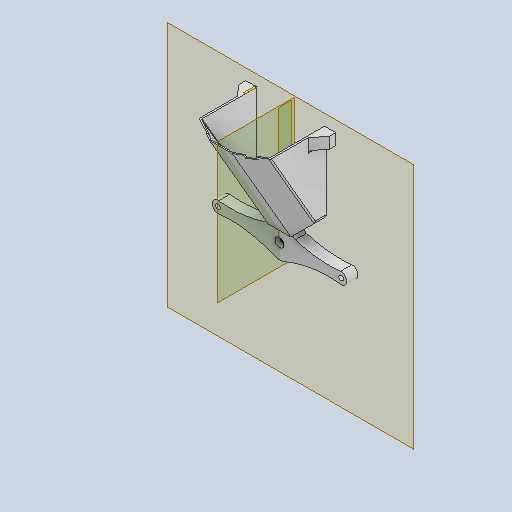
# Autodesk Inventor part: Brida_Rodamiento_Inferior
Saved by Autodesk Inventor 2024 (Build 280153000, 153)
## iProperties
Created: 2024-07-16
Part Number: Brida_Rodamiento_Inferior
Material: Genérico
Document SubType Name: Modeling
Designer: sergi
Density: 1 g/cm^3
Appearance: Valor por defecto
Author: sergi
Autodesk Inventor part; units mm, degrees
ref_plane "YZ Plane" through (0, 0, 0) normal (1, 0, 0) x (0, 1, 0)
ref_plane "XZ Plane" through (0, 0, 0) normal (0, 1, 0) x (-1, 0, 0)
ref_plane "XY Plane" through (0, 0, 0) normal (0, 0, 1) x (1, 0, 0)
sketch "Boceto1" plane through (0, 0, 0) normal (0, 0, 1) x (1, 0, 0)
  circle A0 centre (0, 0) radius 8.25 projected
  arc A1 (-36.7643, -25.9497) -> (36.7643, -25.9497) centre (0, 0) ccw projected
  arc A2 (-35.5756, -20.5396) -> (-36.7643, -25.9497) centre (-33.7006, -23.7872) ccw projected
  line L0 (-35.5756, -20.5396) -> (-15.9099, -9.1856) projected
  arc A3 (-11.2279, -9.9465) -> (-15.9099, -9.1856) centre (-14.0349, -12.4332) ccw projected
  arc A4 (-11.2279, -9.9465) -> (11.2279, -9.9465) centre (0, 0) ccw projected
  arc A5 (15.9099, -9.1856) -> (11.2279, -9.9465) centre (14.0349, -12.4332) ccw projected
  line L1 (15.9099, -9.1856) -> (35.5756, -20.5396) projected
  arc A6 (36.7643, -25.9497) -> (35.5756, -20.5396) centre (33.7006, -23.7872) ccw projected
  line L2 (98, -98) -> (98, 98) projected
  line L3 (98, 98) -> (-98, 98) projected
  line L4 (-98, 98) -> (-98, -98) projected
  line L5 (-98, -98) -> (98, -98) projected
  circle A7 centre (0, 0) radius 4 projected
  line L6 (21.4655, -12.3931) -> (15.9099, -9.1856) projected
  arc A8 (15.9099, -9.1856) -> (11.2279, -9.9465) centre (14.0349, -12.4332) ccw projected
  arc A9 (-11.2279, -9.9465) -> (11.2279, -9.9465) centre (0, 0) ccw projected
  arc A10 (-11.2279, -9.9465) -> (-15.9099, -9.1856) centre (-14.0349, -12.4332) ccw projected
  line L7 (-15.9099, -9.1856) -> (-21.4655, -12.3931) projected
  line L8 (0, 0) -> (-55, 0) construction
  line L9 (0, 0) -> (55, 0) construction
  circle A11 centre (-55, 0) radius 2.1
  circle A12 centre (0, 0) radius 4
  circle A13 centre (-55, 0) radius 5
  circle A14 centre (0, 0) radius 13.4
  circle A15 centre (44.1778, -104.4408) radius 100
  circle A16 centre (-44.1778, -104.4408) radius 100
  arc A17 (0, 14.7284) -> (-5.2203, 12.3413) centre (-44.1778, 104.4408) ccw
  arc A18 (5.2203, 12.3413) -> (0, 14.7284) centre (44.1778, 104.4408) ccw
  line L10 (0, 0) -> (55, 0) construction
  circle A19 centre (55, 0) radius 5
  circle A20 centre (55, 0) radius 2.1
  line L11 (21.4655, -12.3931) -> (21.4655, 21.4655) projected
  line L12 (-21.4655, 21.4655) -> (-21.4655, -12.3931) projected
  line L13 (21.4655, 21.4655) -> (-21.4655, 21.4655) projected
  line L14 (-5.2203, 12.3413) -> (5.2203, 12.3413)
  line L15 (-11.6313, 9.8854) -> (11.6313, 9.8854)
  point P0 (0, 0)
  point P1 (21.8181, -12.5967)
  point P2 (-21.8181, -12.5967)
  point P3 (-11.6313, -9.4678)
  point P4 (-6.1957, 13.6607)
  point P5 (-54.4847, 4.9734)
  point P6 (-54.4847, -4.9734)
  point P7 (-14.9695, -8.8015)
  point P8 (14.9695, -8.8015)
  point P9 (6.1957, 13.6607)
  point P10 (27.9997, -35.2281)
  point P11 (-27.9997, -35.2281)
  point P12 (-11.1255, -10.061)
  point P13 (11.1255, -10.061)
  point P14 (11.2279, -9.9465)
  point P15 (11.2279, -9.9465)
  point P16 (54.4847, -4.9734)
  point P17 (54.4847, 4.9734)
  point P18 (25.5998, 0)
  point P19 (43.9457, 0)
  point P20 (-43.9457, 0)
  point P21 (-25.5998, 0)
  point P22 (-5.2203, -12.3413)
  point P23 (5.2203, -12.3413)
  point P24 (0, 192.7304)
  point P25 (0, 194.1532)
  point P26 (0, -194.1532)
  point P27 (0, -14.7284)
  point P28 (0.5287, -14.9907)
  point P29 (-0.5287, -14.9907)
  dimension "d3" = 180
  dimension "d4" = 4.2
  dimension "d16" = 10
  dimension "d18" = 55
  dimension "d19" = 26.8
  dimension "empalme" = 200
  dimension "d22" = 200
  dimension "d23" = 200
  dimension "d24" = 200
  dimension "d27" = 55
  dimension "d28" = 10
  dimension "d29" = 4.2
  constraints: 10 centre point, 10 end point, 8 point on circle, 8 tangent, 6 coincident, 3 horizontal, 1 collinear, 1 concentric, 1 point on line
  measures "d3" angle of L8 L9
  measures "d4" diameter of A11
  measures "d16" diameter of A13
  measures "d18" distance of L8.start L8.end
  measures "d19" diameter of A14
  measures "empalme" diameter of A15
  measures "d22" diameter of A16
  measures "d23" diameter of A17
  measures "d24" diameter of A18
  measures "d27" distance of L10.start L10.end
  measures "d28" diameter of A19
  measures "d29" diameter of A20
extrude "Extrusión1" add sketch "Boceto1" along normal blind 10 contours A0 | A16 A3 A4 | A4 A3 A16 L12 A17 L15 A14 | A16 A13 A17 L12 | A15 A14 L15 A18 L11 A5 A4 | A4 A5 A15 | A14 L15 | A13 | L11 A18 A19 A15 | A19
sketch "Boceto2" plane through (0, 0, 0) normal (0, 0, -1) x (-1, 0, 0)
  circle A0 centre (0, 0) radius 8.25 projected
  point P0 (0, 0)
extrude "Extrusión2" cut sketch "Boceto2" against normal blind 5
sketch "Boceto3" plane through (0, 0, 5) normal (0, 0, -1) x (-1, 0, 0)
  circle A0 centre (0, 0) radius 5.25 projected
  point P0 (0, 0)
extrude "Extrusión3" cut sketch "Boceto3" against normal blind 0.5
ref_plane "Plano de trabajo1" through (0, 0, 0) normal (0, 0, 1) x (1, 0, 0)
sketch "Boceto4" plane through (0, 0, 0) normal (0, 0, 1) x (1, 0, 0)
  line L0 (-31.8102, 100) -> (-31.8102, 32.4528) projected
  arc A0 (-31.8102, 32.4528) -> (-30.7558, 29.9072) centre (-28.2102, 32.4528) ccw projected
  line L1 (-30.7558, 29.9072) -> (-10.7339, 9.8854) projected
  line L2 (10.7339, 9.8854) -> (10.7339, 100) projected
  line L3 (30.7558, 29.9072) -> (30.7558, 100) projected
  line L4 (30.7558, 29.9072) -> (10.7339, 9.8854) projected
  line L5 (30.7558, 29.9072) -> (30.7558, 100) projected
  line L6 (-30.2102, 32.4528) -> (-30.2102, 100) projected
  arc A1 (-30.2102, 32.4528) -> (-29.6244, 31.0386) centre (-28.2102, 32.4528) ccw projected
  line L7 (-9.8759, 11.2901) -> (-29.6244, 31.0386) projected
  line L8 (9.8759, 11.2901) -> (-9.8759, 11.2901) projected
  line L9 (11.6313, 9.8854) -> (-11.6313, 9.8854) projected
  line L10 (29.6244, 31.0386) -> (9.8759, 11.2901) projected
  arc A2 (29.6244, 31.0386) -> (30.2102, 32.4528) centre (28.2102, 32.4528) ccw projected
  line L11 (30.2102, 100) -> (30.2102, 32.4528) projected
  line L12 (100, 100) -> (-100, 100) projected
  line L13 (31.8102, 32.4528) -> (31.8102, 100) projected
  arc A3 (30.7558, 29.9072) -> (31.8102, 32.4528) centre (28.2102, 32.4528) ccw projected
  line L14 (11.6313, 9.8854) -> (11.6313, 10.7827)
  line L15 (-11.6313, 9.8854) -> (-11.6313, 10.7827)
  point P0 (0, 0)
  point P1 (10.7339, 12.1481)
  constraints: 4 end point, 2 point on line, 1 parallel, 1 vertical
extrude "Extrusión4" add sketch "Boceto4" along normal up to surface (10 mm away) contours L12 L6 A1 L7 L8 L10 L2 L9 L1 A0 L0 | L1 L9 L15 | L10 A2 L11 L12 L3 L4 L2 | L4 L14 L9 | L12 L13 A3 L3
fillet "Empalme2" radius 2 4 edges at (-11.6313, 9.8854, 5) (-11.6313, 10.7827, 5) (11.6313, 9.8854, 5) (11.6313, 10.7827, 5)
sketch "Boceto5" plane through (0, 0, 10) normal (0, 0, 1) x (1, 0, 0)
  line L0 (-10.1386, 9.2901) -> (-30.7558, 29.9072)
  arc A0 (-31.8102, 32.4528) -> (-30.7558, 29.9072) centre (-28.2102, 32.4528) ccw projected
  arc A1 (-30.2102, 32.4528) -> (-29.6244, 31.0386) centre (-28.2102, 32.4528) ccw projected
  line L1 (-29.6244, 31.0386) -> (-9.8759, 11.2901) projected
  line L2 (-9.8759, 11.2901) -> (9.8759, 11.2901) projected
  line L3 (9.8759, 11.2901) -> (29.6244, 31.0386) projected
  line L4 (30.7558, 29.9072) -> (10.1386, 9.2901)
  arc A2 (30.7558, 29.9072) -> (31.8102, 32.4528) centre (28.2102, 32.4528) ccw projected
  line L5 (-103, 100) -> (100, 100) projected
  arc A3 (-54.4847, 4.9734) -> (-11.6313, 9.8854) centre (-44.1778, 104.4408) ccw projected
  arc A4 (-54.4847, 4.9734) -> (-11.6313, 9.8854) centre (-44.1778, 104.4408) ccw projected
  arc A5 (13.4151, 9.2901) -> (54.4847, 4.9734) centre (44.1778, 104.4408) ccw
  line L6 (11.6313, 10.7827) -> (11.6313, 9.8854) projected
  line L7 (-11.6313, 9.8854) -> (-11.6313, 10.7827) projected
  arc A6 (-54.4847, 4.9734) -> (-14.0645, 9.0826) centre (-44.1778, 104.4408) ccw projected
  arc A7 (-54.4847, 4.9734) -> (-54.4847, -4.9734) centre (-55, 0) ccw projected
  arc A8 (-5.2203, -12.3413) -> (-54.4847, -4.9734) centre (-44.1778, -104.4408) ccw projected
  arc A9 (-5.2203, -12.3413) -> (5.2203, -12.3413) centre (0, 0) ccw projected
  arc A10 (54.4847, -4.9734) -> (5.2203, -12.3413) centre (44.1778, -104.4408) ccw projected
  arc A11 (54.4847, -4.9734) -> (54.4847, 4.9734) centre (55, 0) ccw projected
  arc A12 (14.0645, 9.0826) -> (54.4847, 4.9734) centre (44.1778, 104.4408) ccw projected
  circle A13 centre (0, 0) radius 4 projected
  line L8 (-14.0645, 9.0826) -> (-14.0158, 9.0987)
  line L9 (0, 11.2901) -> (0, 9.2901)
  line L10 (0, 9.2901) -> (-13.4151, 9.2901)
  line L11 (0, 9.2901) -> (13.4151, 9.2901)
  line L12 (30.7558, 29.9072) -> (13.2525, 12.404) projected
  arc A14 (30.7558, 29.9072) -> (31.8102, 32.4528) centre (28.2102, 32.4528) ccw projected
  line L13 (31.8102, 100) -> (31.8102, 32.4528) projected
  line L14 (30.2102, 100) -> (31.8102, 100) projected
  line L15 (30.2102, 32.4528) -> (30.2102, 100) projected
  arc A15 (29.6244, 31.0386) -> (30.2102, 32.4528) centre (28.2102, 32.4528) ccw projected
  line L16 (9.8759, 11.2901) -> (29.6244, 31.0386) projected
  line L17 (-9.8759, 11.2901) -> (9.8759, 11.2901) projected
  line L18 (-29.6244, 31.0386) -> (-9.8759, 11.2901) projected
  arc A16 (-30.2102, 32.4528) -> (-29.6244, 31.0386) centre (-28.2102, 32.4528) ccw projected
  line L19 (-30.2102, 100) -> (-30.2102, 32.4528) projected
  line L20 (-31.8102, 100) -> (-30.2102, 100) projected
  line L21 (-31.8102, 32.4528) -> (-31.8102, 100) projected
  arc A17 (-31.8102, 32.4528) -> (-30.7558, 29.9072) centre (-28.2102, 32.4528) ccw projected
  line L22 (-13.2525, 12.404) -> (-30.7558, 29.9072) projected
  arc A18 (-14.0645, 9.0826) -> (-13.2525, 12.404) centre (-14.6667, 10.9898) ccw projected
  arc A19 (13.2525, 12.404) -> (14.0645, 9.0826) centre (14.6667, 10.9898) ccw projected
  point P0 (0, 0)
  point P1 (-31.8102, 100)
  point P2 (-30.2102, 100)
  point P3 (30.2102, 100)
  point P4 (31.8102, 100)
  point P5 (-31.8102, 32.4528)
  dimension "d59" = 2
  constraints: 12 end point, 4 point on circle, 2 point on line, 1 centre point, 1 horizontal, 1 perpendicular
  measures "d59" distance of L9.start L9.end
ref_plane "Plano de trabajo2" through (0, 32.4528, 0) normal (-1, 0, 0) x (0, 0, 1)
sketch "Boceto6" plane through (0, 32.4528, 0) normal (-1, 0, 0) x (0, 0, 1)
  line L0 (10, -23.1627) -> (81, 99.8129)
  point P0 (10, 67.5472)
  constraints: 2 end point
sweep "Barrido1" add profiles "Boceto5" path "Boceto6" keep normal constant yes contours L0 A0 L21 L5 L19 A1 L1 L2 L9 L10 | L9 L2 L3 A15 L15 L5 L13 A2 L4 L11
ref_plane "Plano de trabajo3" through (-31.8102, 100, 0) normal (0, 1, 0) x (1, 0, 0)
split "Dividir1" plane through (-31.8102, 100, 0) removes the side toward (0, 1, 0)
sketch "Boceto7" plane through (-31.8102, 32.4528, 0) normal (-1, 0, 0) x (0, 0, 1)
  line L0 (0, 67.5472) -> (48.9984, 67.5472) projected
  line L1 (0, 67.5472) -> (0, 0) projected
  line L2 (0, 0) -> (10, 0) projected
  line L3 (0, 67.5472) -> (16, 67.5472)
  line L4 (16, 67.5472) -> (16, 57.5472)
  line L5 (16, 57.5472) -> (0, 57.5472)
  line L6 (0, 57.5472) -> (0, 67.5472)
  line L7 (10, 0) -> (48.9984, 67.5472) projected
  point P0 (0, -32.4528)
  point P1 (0, 57.5472)
  point P2 (16, 67.5472)
  point P3 (16, 67.5472)
  dimension "d41" = 10
  dimension "d56" = 16
  constraints: 8 end point, 2 parallel, 1 horizontal, 1 perpendicular
  measures "d41" distance of L3.end L4.end
  measures "d56" distance of L4.end L5.end
extrude "Extrusión5" add sketch "Boceto7" along normal blind 8.4 contours L0 L4 L5 L1
chamfer "Chaflán2" distance 10 distance2 8.4 1 edges at (-40.2102, 95, 16) measured on face at (-40.2102, 95, 15.5)
sketch "Boceto8" plane through (0, 0, 0) normal (0, 0, -1) x (-1, 0, 0)
  line L0 (30.2102, 100) -> (-31.8102, 100) projected
  line L1 (30.2102, 32.4528) -> (30.2102, 100) projected
  line L2 (40.2102, 100) -> (40.2102, 90) projected
  line L3 (-98, 100) -> (100, 100) projected
  line L4 (31.8102, 90) -> (40.2102, 90) projected
  line L5 (31.8102, 90) -> (31.8102, 32.4528) projected
  circle A0 centre (35, 95) radius 2.1
  point P0 (0, 0)
  point P1 (25.2102, 95)
  point P2 (31.8102, 100)
  dimension "d47" = 5
  dimension "d55" = 5
  dimension "d62" = 4.2
  constraints: 1 centre point
  measures "d47" distance from line of L0 point (25.21, 95)
  measures "d55" distance from line of L1 point (25.21, 95)
  measures "d62" diameter of A0
hole "Agujero1" at (-35, 95, 0) direction (0, 0, 1) diameter 4.2 depth 4
ref_plane "Plano de trabajo4" through (0, 32.4528, 0) normal (-1, 0, 0) x (0, 0, 1)
mirror "Simetría1" about plane through (0, 32.4528, 0) normal (-1, 0, 0) of "Extrusión5", "Chaflán2", "Agujero1"
fillet "Empalme1" radius 2 4 edges at (-31.8102, 90, 16) (-31.8102, 90, 8) (31.8102, 90, 16) (31.8102, 90, 8)
sketch "Boceto9" plane through (-10.1386, 100, 62.3714) normal (0, 1, 0) x (1, 0, 0)
  line L0 (-89.8614, 115.3714) -> (-92.8614, 115.3714) projected
  line L1 (-92.8614, 115.3714) -> (-92.8614, 90.3714) projected
  line L2 (-92.8614, 90.3714) -> (-89.8614, 90.3714) projected
  line L3 (-89.8614, 90.3714) -> (-89.8614, 65.3714) projected
  line L4 (-89.8614, 65.3714) -> (-92.8614, 65.3714) projected
  line L5 (-92.8614, 65.3714) -> (-92.8614, 40.3714) projected
  line L6 (-92.8614, 40.3714) -> (-89.8614, 40.3714) projected
  line L7 (-89.8614, 40.3714) -> (-89.8614, 15.3714) projected
  line L8 (-89.8614, 15.3714) -> (-92.8614, 15.3714) projected
  line L9 (-92.8614, 15.3714) -> (-92.8614, -9.6286) projected
  line L10 (-92.8614, -9.6286) -> (-89.8614, -9.6286) projected
  line L11 (-89.8614, -9.6286) -> (-89.8614, -34.6286) projected
  line L12 (-89.8614, -34.6286) -> (-92.8614, -34.6286) projected
  line L13 (-92.8614, -34.6286) -> (-92.8614, -59.6286) projected
  line L14 (-92.8614, -59.6286) -> (-89.8614, -59.6286) projected
  line L15 (-89.8614, -59.6286) -> (-89.8614, -84.6286) projected
  line L16 (-89.8614, -84.6286) -> (-14.8614, -84.6286) projected
  line L17 (113.1386, -84.6286) -> (113.1386, -59.6286) projected
  line L18 (113.1386, -59.6286) -> (110.1386, -59.6286) projected
  line L19 (110.1386, -59.6286) -> (110.1386, -34.6286) projected
  line L20 (110.1386, -34.6286) -> (113.1386, -34.6286) projected
  line L21 (113.1386, -34.6286) -> (113.1386, -9.6286) projected
  line L22 (113.1386, -9.6286) -> (110.1386, -9.6286) projected
  line L23 (110.1386, -9.6286) -> (110.1386, 15.3714) projected
  line L24 (110.1386, 15.3714) -> (113.1386, 15.3714) projected
  line L25 (113.1386, 15.3714) -> (113.1386, 40.3714) projected
  line L26 (113.1386, 40.3714) -> (110.1386, 40.3714) projected
  line L27 (110.1386, 40.3714) -> (110.1386, 65.3714) projected
  line L28 (110.1386, 65.3714) -> (113.1386, 65.3714) projected
  line L29 (113.1386, 65.3714) -> (113.1386, 90.3714) projected
  line L30 (113.1386, 90.3714) -> (110.1386, 90.3714) projected
  line L31 (110.1386, 90.3714) -> (110.1386, 115.3714) projected
  line L32 (110.1386, 115.3714) -> (113.1386, 115.3714) projected
  line L33 (113.1386, 115.3714) -> (113.1386, 140.3714) projected
  line L34 (113.1386, 140.3714) -> (110.1386, 140.3714) projected
  line L35 (110.1386, 140.3714) -> (110.1386, 165.3714) projected
  line L36 (110.1386, 165.3714) -> (-92.8614, 165.3714) projected
  line L37 (-92.8614, 165.3714) -> (-92.8614, 140.3714) projected
  line L38 (-92.8614, 140.3714) -> (-89.8614, 140.3714) projected
  line L39 (-89.8614, 140.3714) -> (-89.8614, 115.3714) projected
  circle A0 centre (-39.8614, 150.3714) radius 1.75 projected
  circle A1 centre (60.1386, 150.3714) radius 1.75 projected
  circle A2 centre (60.1386, -72.6286) radius 1.5 projected
  circle A3 centre (-39.8614, -72.6286) radius 1.5 projected
  circle A4 centre (-39.8614, 50.3714) radius 1.5 projected
  circle A5 centre (60.1386, 50.3714) radius 1.5 projected
  line L40 (31.6817, 7.8907) -> (31.6817, -2.9753) projected
  line L41 (31.6817, -2.9753) -> (28.6817, -2.9753) projected
  line L42 (28.6817, -2.9753) -> (28.6817, 6.1587) projected
  line L43 (28.6817, 6.1587) -> (20.0145, 1.1547) projected
  line L44 (20.0145, 1.1547) -> (0.2627, 1.1547) projected
  line L45 (0.2627, 1.1547) -> (-8.4044, 6.1587) projected
  line L46 (-8.4044, 6.1587) -> (-8.4044, -2.9753) projected
  line L47 (-8.4044, -2.9753) -> (-11.4044, -2.9753) projected
  line L48 (-11.4044, -2.9753) -> (-11.4044, 7.8907) projected
  line L49 (-11.4044, 7.8907) -> (-19.4858, 12.5565) projected
  ellipse E0 centre (-18.0715, 13.373) end of major axis (-16.0715, 13.373) minor radius 1.1547 (-20.0715, 13.373) -> (-19.4858, 12.5565) ccw projected
  line L50 (-20.0715, 13.373) -> (-20.0715, 23.373) projected
  line L51 (-20.0715, 23.373) -> (40.3488, 23.373) projected
  line L52 (40.3488, 23.373) -> (40.3488, 13.373) projected
  ellipse E1 centre (38.3488, 13.373) end of major axis (40.3488, 13.373) minor radius 1.1547 (39.763, 12.5565) -> (40.3488, 13.373) ccw projected
  line L53 (39.763, 12.5565) -> (31.6817, 7.8907) projected
  line L54 (-6.4044, -4.9753) -> (-6.4044, 2.6946)
  line L55 (-6.4044, 2.6946) -> (-0.2732, -0.8453)
  line L56 (-0.2732, -0.8453) -> (20.5504, -0.8453)
  line L57 (20.5504, -0.8453) -> (26.6817, 2.6946)
  line L58 (26.6817, 2.6946) -> (26.6817, -4.9753)
  line L59 (26.6817, -4.9753) -> (33.6817, -4.9753)
  line L60 (33.6817, -4.9753) -> (33.6817, 6.736)
  line L61 (33.6817, 6.736) -> (40.763, 10.8244)
  line L62 (42.3488, 13.373) -> (42.3488, 25.373)
  line L63 (42.3488, 25.373) -> (-22.0715, 25.373)
  line L64 (-22.0715, 25.373) -> (-22.0715, 13.373)
  line L65 (-20.4858, 10.8244) -> (-13.4044, 6.736)
  line L66 (-13.4044, 6.736) -> (-13.4044, -4.9753)
  line L67 (-13.4044, -4.9753) -> (-6.4044, -4.9753)
  line L68 (-13.4044, 6.736) -> (-13.4044, 14)
  line L69 (-13.4044, 14) -> (-6.4044, 14)
  line L70 (-6.4044, 14) -> (-6.4044, 2.6946)
  line L71 (26.6817, -4.9753) -> (33.6817, -4.9753)
  line L72 (33.6817, -4.9753) -> (33.6817, 14)
  line L73 (33.6817, 14) -> (26.6817, 14)
  line L74 (26.6817, 14) -> (26.6817, -4.9753)
  line L75 (32.1386, -84.6286) -> (32.1386, -69.6286) projected
  line L76 (32.1386, -69.6286) -> (35.1386, -69.6286) projected
  line L77 (35.1386, -69.6286) -> (35.1386, -84.6286) projected
  line L78 (35.1386, -84.6286) -> (113.1386, -84.6286) projected
  line L79 (-14.8614, -84.6286) -> (-14.8614, -69.6286) projected
  line L80 (-14.8614, -69.6286) -> (-11.8614, -69.6286) projected
  line L81 (-11.8614, -69.6286) -> (-11.8614, -84.6286) projected
  line L82 (2.6386, -84.6286) -> (2.6386, -74.6286) projected
  line L83 (2.6386, -74.6286) -> (17.6386, -74.6286) projected
  line L84 (17.6386, -74.6286) -> (17.6386, -84.6286) projected
  line L85 (17.6386, -84.6286) -> (32.1386, -84.6286) projected
  line L86 (-11.8614, -84.6286) -> (2.6386, -84.6286) projected
  spline S0 degree 4 poles (40.763, 10.8245) (41.0721, 11.0028) (41.3594, 11.2191) (41.9199, 11.7841) (42.2561, 12.5129) (42.3487, 12.9428) (42.3488, 13.373) knots 0 0 0 0 0 0.453465 0.453465 1 1 1 1 1
  spline S1 degree 4 poles (-22.0716, 13.373) (-22.0714, 12.9428) (-21.9789, 12.5129) (-21.6426, 11.7841) (-21.0821, 11.2191) (-20.7948, 11.0028) (-20.4858, 10.8245) knots 0 0 0 0 0 0.546535 0.546535 1 1 1 1 1
  point P0 (10.1386, 62.3714)
  point P1 (26.6817, 2.6946)
  point P2 (33.6817, 4.333)
  point P3 (33.6817, 4.736)
  point P4 (26.6817, 2.6946)
  point P5 (33.6817, 6.736)
  dimension "d63" = 2
  constraints: 42 end point, 6 parallel, 3 perpendicular, 1 horizontal, 1 vertical, 19 other
  measures "d63" distance between parallel lines of L46 L54
extrude "Extrusión6" cut sketch "Boceto9" against normal blind 3 contours L53 L72 L60 L59 L58 L74 L43 L42 L41 L40 | L40 L41 L42 L43 L74 L73 L72 L53 | L70 L54 L67 L66 L68 L49 L48 L47 L46 L45 | L45 L46 L47 L48 L49 L68 L69 L70
equation "\"d22\" = empalme"
equation "\"d23\" = empalme"
equation "\"d24\" = empalme"
